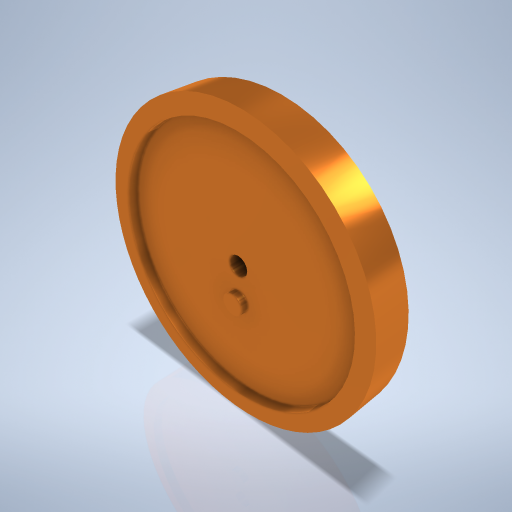
# Autodesk Inventor part: rad
Saved by Autodesk Inventor 2024.2 (Build 282272000, 272)
## iProperties
Created: 2024-05-05
Part Number: rad
Material: Gold
Document SubType Name: Modeling
Designer: Fabri
Density: 19.3 g/cm^3
Appearance: Metall - 1600F (heiß)
Author: Fabri
Autodesk Inventor part; units mm, degrees
ref_plane "YZ Plane" through (0, 0, 0) normal (1, 0, 0) x (0, 1, 0)
ref_plane "XZ Plane" through (0, 0, 0) normal (0, 1, 0) x (-1, 0, 0)
ref_plane "XY Plane" through (0, 0, 0) normal (0, 0, 1) x (1, 0, 0)
sketch "Skizze1" plane through (0, 0, 0) normal (0, 1, 0) x (-1, 0, 0)
  circle A0 centre (0, 0) radius 200
  dimension "d0" = 400
  constraints: 1 centre point, 1 coincident
  measures "d0" diameter of A0
extrude "Extrusion1" add sketch "Skizze1" along normal mid plane 50
sketch "Skizze2" plane through (0, 25, 0) normal (0, 1, 0) x (1, 0, 0)
  circle A0 centre (0, 0) radius 200 projected
  constraints: 1 coincident
hole "Bohrung1" at (0, 25, 0) direction (0, -1, 0) diameter 350 depth 15
mirror "Spiegeln1" about plane through (0, 0, 0) normal (0, 1, 0) of "Bohrung1"
sketch "Skizze3" plane through (0, 10, 0) normal (0, 1, 0) x (1, 0, 0)
  circle A0 centre (0, 0) radius 75
  dimension "d11" = 150
  constraints: 1 centre point, 1 coincident
  measures "d11" diameter of A0
extrude "Extrusion2" add sketch "Skizze3" along normal blind 50
sketch "Skizze4" plane through (0, 60, 0) normal (0, 1, 0) x (1, 0, 0)
  circle A0 centre (0, 0) radius 75 projected
  constraints: 1 coincident
hole "Bohrung2" at (0, 60, 0) direction (0, -1, 0) diameter 28 depth 70
sketch "Skizze7" plane through (0, -10, 0) normal (0, -1, 0) x (1, 0, 0)
  circle A0 centre (0, -48.21) radius 15
  point P0 (0, 0)
  dimension "d46" = 30
  dimension "d50" = 48.21
  constraints: 1 centre point, 1 vertical alignment
  measures "d46" diameter of A0
  measures "d50" distance of point (0, 0) A0.centre
extrude "Extrusion3" add sketch "Skizze7" along normal blind 10
